2.5mm_bottom_thick (Autodesk Fusion 360 design; units mm, degrees)
Autodesk Fusion 360 part; units mm, degrees
note: some values were not read from the file. Set by a fixed rule: which sketch regions a step uses.
sketch "Sketch7" plane through (0, 0, 0) normal (1, 0, 0) x (0, 1, 0)
  line L0 (0, 0) -> (1, 0)
  line L1 (-2.9, 0.5625) -> (-2.9, 0.4625)
  line L2 (-2.9, 0.4625) -> (0, 0.4625)
  line L3 (-2.6, 0.6125) -> (-2.9, 0.5625)
  line L4 (0.0797, 1.1059) -> (1, 0.9437)
  line L5 (1, 0.9437) -> (1, 0)
  line L6 (-2.6, 0.6125) -> (-1.45, 0.6125)
  line L7 (-1.45, 0.6125) -> (-1.45, 0.5625)
  line L8 (-1.45, 0.5625) -> (-0.65, 0.5625)
  line L9 (-0.65, 0.5625) -> (-0.65, 0.6125)
  line L10 (-0.65, 0.6125) -> (0, 0.6125)
  line L11 (0.0079, 1.0394) -> (0.05, 0.6125)
  line L12 (0.05, 0.6125) -> (0, 0.6125)
  line L13 (0, 0.4625) -> (0, 0)
  line L14 (0.0797, 1.1059) -> (0.0079, 1.0394)
  point P0 (0, 1.12)
  dimension "d25" = 0.05
  dimension "d26" = 0.3
  dimension "d27" = 1.12
  dimension "d29" = 1
  dimension "d30" = 100
  dimension "d31" = 0.05
  dimension "d32" = 0.8
  dimension "d33" = 1.45
  dimension "d34" = 3.9
  dimension "d36" = 0.4625
  dimension "d37" = 0.6125
  dimension "d48" = 0.05
  dimension "d49" = 0.081
  dimension "d50" = 0.081
  constraint horizontal L0
  constraint coincident L0.start L13.end
  constraint horizontal L6
  constraint perpendicular L6 L7
  constraint perpendicular L7 L8
  constraint perpendicular L8 L9
  constraint collinear L6 L10
  constraint perpendicular L0 L13
  constraint vertical P0 L2.end
  constraint horizontal L12
  constraint horizontal L2
  constraint vertical L5
  constraint vertical L2.end L10.end
  constraint coincident P0 L4
  constraint coincident P0 L11
  measures "d25" vertical distance of L1.start L3.start
  measures "d26" horizontal distance of L1.start L3.start
  measures "d27" distance of L0.start P0
  measures "d29" distance of L0.start L0.end
  measures "d30" angle of L4 L5
  measures "d31" distance of L8.end L9.end
  measures "d32" distance of L7.end L8.end
  measures "d33" distance of L1 L6.end
  measures "d34" distance of L1 L5
  measures "d36" distance of L0.start L2
  measures "d37" distance of L0.start L10
  measures "d48" distance of L10.end L11.end
  measures "d49" distance of P0 L4.start
  measures "d50" distance of P0 L11.start
revolve "Revolve2" add sketch "Sketch7" angle 360 about axis through (0, 0, 0) along (0, 1, 0)
sketch "Sketch8" plane through (0, -2.9, 0) normal (0, -1, 0) x (1, 0, 0)
  circle A0 centre (0, 0) radius 0.4625
  circle A1 centre (0, 0) radius 0.5625
  circle A2 centre (0, 0.64) radius 0.05
  dimension "d38" = 0.1
  dimension "d41" = 0.64
  measures "d38" diameter of A2
  measures "d41" distance of A0.centre A2.centre
move_body "Move1" bodies 1 to x (0.999879, 0.015553, 0.000062) y (-0.015553, 0.999848, 0.007918) z (0.000062, -0.007918, 0.999969) at (-0.0315, -0.0003, 0.016)
move_body "Move2" bodies 1 to x (1, 0, 0) y (0, 0, 1) z (0, -1, 0) at (0, 0, 0)
equation "d27 = 2.240 mm / 2"
equation "d36 = ( 0.925 / 2 ) * 1 mm"
equation "d37 = var / 2"
equation "var = 1.225 mm"
equation "d50 = d49"
